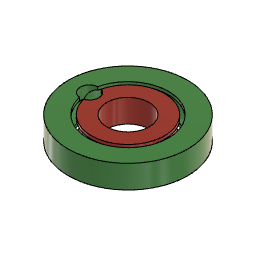
No Cage (Autodesk Fusion 360 design; units mm, degrees)
Autodesk Fusion 360 part; units mm, degrees
sketch "Sketch4" plane through (0, 0, 6) normal (0, 0, 1) x (-1, 0, 0)
  circle A0 centre (0, 0) radius 10.5
  circle A1 centre (0, 0) radius 15.5
  circle A2 centre (0, 0) radius 10 construction
  circle A3 centre (10, 0) radius 2.4
  dimension "d1" = 4.8
  constraint coincident A2 A3.centre
  measures "d1" diameter of A3
sketch "Sketch1" plane through (0, 0, 0) normal (0, 0, 1) x (1, 0, 0)
  circle A0 centre (0, 0) radius 5.5
  circle A1 centre (0, 0) radius 9.5
  circle A2 centre (0, 0) radius 10 construction
  circle A3 centre (0, 0) radius 10.5
  circle A4 centre (0, 0) radius 15.5
  dimension "Gap" = 0.5
  dimension "d4" = 0.5
  dimension "bearingPCD" = 20
  dimension "pcdToID" = 4.5
  dimension "pcdToOD" = 5.5
  constraint coincident A0.centre A1.centre
  constraint concentric A2 A3
  constraint concentric A0 A4
  measures "Gap" distance of A1 A2
  measures "d4" distance of A2 A3
  measures "bearingPCD" diameter of A2
  measures "pcdToID" distance of A0 A2
  measures "pcdToOD" distance of A2 A4
extrude "Extrude1" add sketch "Sketch1" along normal blind 6 makes body 1 at (9.4882, -0.4735, 4) makes body 2 at (15.4807, -0.7726, 4)
sketch "Sketch2" plane through (0, 0, 0) normal (0, 1, 0) x (1, 0, 0)
  line L0 (-10, 0) -> (10, 0)
  line L1 (10, 0) -> (10, -3) construction
  circle A0 centre (10, -3) radius 2.25
  line L2 (10, 0) -> (10, -5.25)
  dimension "d9" = 3
  dimension "balldiameter" = 4.5
  constraint coincident L0.end L1.start
  constraint perpendicular L0 L1
  constraint coincident L1.end A0.centre
  constraint coincident A0 L2.end
  constraint perpendicular L0 L2
  measures "d9" distance of L0.end L1.end
  measures "balldiameter" diameter of A0
revolve "Revolve1" cut sketch "Sketch2" angle 360 about axis through (0, 0, 1.75) along (0, 0, 1) bodies 1 2
ref_plane "WorkPlane1" through (0, 0, 5) normal (0, 0, 1) x (1, 0, 0)
split "Split1" by plane through (0, 0, 5) normal (0, 0, 1) bodies 2 makes body 3 at (13.7756, -0.7701, 6)
sketch "Sketch3" plane through (0, 0, 5) normal (0, 0, 1) x (-1, 0, 0)
  circle A0 centre (0, 0) radius 11.0308
  circle A1 centre (0, 0) radius 15.5
  circle A2 centre (0, 0) radius 14
  circle A3 centre (0, 0) radius 15.5
  dimension "d21" = 1.5
  constraint coincident A0.centre A1.centre
  measures "d21" distance of A2 A3
extrude "Extrude2" cut sketch "Sketch3" against normal blind 2 contours A1 A3 bodies 2
extrude "Extrude3" add sketch "Sketch3" against normal blind 2 contours A1 A3 bodies 3
revolve "Revolve1'" add sketch "Sketch2" angle 360 about axis through (10, 0, 0) along (0, 0, 1) separate body contours A0 L2 picked at (10.6309, -2.5945) makes body 4 in component "Balls"
pattern_circular "C-Pattern1" count 40 over 360 about axis through (0, 0, 1.75) along (0, 0, 1) of bodies 4 makes body 5 at (8.473, 3.298, 2.7063) makes body 6 at (7.8528, 4.5828, 2.7063) makes body 7 at (8.7933, 2.3122, 2.7063) makes body 8 at (8.3233, 3.6593, 2.7063) makes body 9 at (7.6484, 4.9163, 2.7063) makes body 10 at (8.0964, 7.857, 2.7063) makes body 11 at (6.7676, 9.0268, 2.7063) makes body 12 at (0.9082, 9.0468, 2.7063) makes body 13 at (3.298, 8.473, 2.7063) makes body 14 at (-1.9319, 11.1154, 2.7063) makes body 15 at (0.1693, 11.2807, 2.7063) makes body 16 at (-4.5828, 7.8528, 2.7063) makes body 17 at (-2.3122, 8.7933, 2.7063) makes body 18 at (-3.6593, 8.3233, 2.7063) makes body 19 at (-4.9163, 7.6484, 2.7063) makes body 20 at (-8.3233, 3.6593, 2.7063) makes body 21 at (-9.0268, 6.7676, 2.7063) makes body 22 at (-7.8528, 4.5828, 2.7063) makes body 23 at (-9.0775, -0.5182, 2.7063) makes body 24 at (-8.8846, 1.9319, 2.7063) makes body 25 at (-11.2807, 0.1693, 2.7063) makes body 26 at (-9.9744, -5.2722, 2.7063) makes body 27 at (-9.0268, -6.7676, 2.7063) makes body 28 at (-8.3233, -3.6593, 2.7063) makes body 29 at (-7.6484, -4.9163, 2.7063) makes body 30 at (-3.6593, -8.3233, 2.7063) makes body 31 at (-5.7549, -7.0392, 2.7063) makes body 32 at (-0.9082, -9.0468, 2.7063) makes body 33 at (-3.298, -8.473, 2.7063) makes body 34 at (-1.9319, -8.8846, 2.7063) makes body 35 at (-0.1693, -11.2807, 2.7063) makes body 36 at (1.5975, -11.1683, 2.7063) makes body 37 at (6.7676, -9.0268, 2.7063) makes body 38 at (4.9705, -10.1281, 2.7063) makes body 39 at (4.9163, -7.6484, 2.7063) makes body 40 at (8.3233, -3.6593, 2.7063) makes body 41 at (7.0392, -5.7549, 2.7063) makes body 42 at (7.8528, -4.5828, 2.7063) makes body 43 at (8.473, -3.298, 2.7063) in component "Balls"
move_face "OffsetFaces2" offset -0.01 5 faces at (12.0992, -0.6038, 2.2303) (-7.0845, -9.8539, 3.7064) (-13.9304, 1.3939, 4.3333) (9.3796, 0.4681, 0.8339) (10.9199, 1.0927, 5.0281) on bodies 1 2 3
extrude "Extrude4" cut sketch "Sketch4" against normal blind 3 contours A0 A3 | A0 A3 picked at (9.5749, -0.5508) picked at (11.0884, -0.5005) bodies 1 3 2
combine "Combine1" operation add target body 3 tool bodies 2
component "Balls" placed x (1, 0, 0) y (0, 1, 0) z (0, 0, 1) at (0, 0, 0)
equation "d4 = Gap"
equation "height = 6 mm"
equation "d9 = height / 2"
equation "offset = -0.01 mm"
equation "d48 = -height / 2"
equation "d1 = balldiameter + 0.3 mm"
